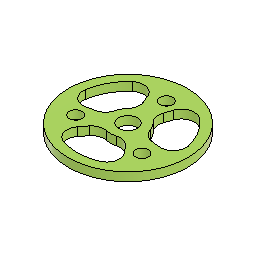
电机2312s磁编码器d4x2定位架 v1 (Autodesk Fusion 360 design; units mm, degrees)
Autodesk Fusion 360 part; units mm, degrees
sketch "草图1" plane through (0, 0, 0) normal (0, 0, 1) x (1, 0, 0)
  circle A0 centre (0, 0) radius 14.1
  line L0 (0, 9.064) -> (-7.85, -4.5326)
  line L1 (-7.85, -4.5326) -> (7.85, -4.5326)
  line L2 (7.85, -4.5326) -> (0, 9.064)
  line L3 (0, 9.064) -> (15.7, 9.064) construction
  circle A1 centre (0, 9.064) radius 1.5
  circle A2 centre (-7.85, -4.5326) radius 1.5
  circle A3 centre (7.85, -4.5326) radius 1.5
  point P0 (0, -0.0004)
  dimension "d1" = 28.2
  dimension "d2" = 15.7
  dimension "d3" = 120
  dimension "d4" = 9.064
  dimension "d5" = 3
  dimension "d6" = 3
  dimension "d7" = 3
  constraint coincident A0.centre origin
  constraint horizontal L3
  constraint coincident L0.start L2.end
  constraint coincident L0.end L1.start
  constraint coincident L1.end L2.start
  measures "d1" diameter of A0
  measures "d2" distance of L0.start L0.end
  measures "d3" angle of L0 L3
  measures "d4" distance of A0.centre L0.start
  measures "d5" diameter of A1
  measures "d6" diameter of A2
  measures "d7" diameter of A3
extrude "拉伸1" add sketch "草图1" along normal blind 2 contours A0 | L0 L1 L2 A1 A2 A3
sketch "草图2" plane through (0, 0, 2) normal (0, 0, 1) x (-1, 0, 0)
  circle A0 centre (7.85, 4.5326) radius 1.5
  circle A1 centre (-7.85, 4.5326) radius 1.5
  circle A2 centre (0, -9.064) radius 1.5
  circle A3 centre (0, 0) radius 14.1
  circle A4 centre (0, 0) radius 2.2
  circle A5 centre (0, 0) radius 12
  circle A6 centre (0, 0) radius 4.2
  line L0 (0, 0) -> (4.5287, -11.1127)
  line L1 (0, 0) -> (11.7731, 2.3225)
  line L2 (0, 0) -> (7.3595, 9.4783)
  line L3 (0, 0) -> (-7.8979, 9.0345)
  line L4 (0, 0) -> (-11.8882, 1.6344)
  line L5 (0, 0) -> (-3.8752, -11.3571)
  dimension "d10" = 4.4
  dimension "d13" = 24
  dimension "d14" = 8.4
  dimension "d16" = 360
  constraint concentric A3 A4
  constraint concentric A4 A5
  constraint concentric A5 A6
  constraint coincident A3.centre A4.centre
  constraint coincident A5 L0.end
  constraint coincident A5 L1.end
  measures "d10" diameter of A4
  measures "d13" diameter of A5
  measures "d14" diameter of A6
extrude "拉伸2" cut sketch "草图2" against normal blind 8 contours A4 L0 L1 | A4 L1 L2 | A4 L0 L5 | A4 L2 L3 | A4 L3 L4 | A4 L4 L5 | A5 A6 L0 L1 | A5 A6 L2 L3 | A5 A6 L4 L5
fillet "圆角1" radius 3 12 edges at (-1.585, 3.8894, 1) (-4.1206, -0.8129, 1) (-2.5758, -3.3174, 1) (2.7643, -3.1621, 1) (4.1609, -0.572, 1) (1.3563, 3.975, 1) (3.8752, 11.3571, 1) (11.8882, -1.6344, 1) (-4.5287, 11.1127, 1) (-11.7731, -2.3225, 1) (-7.3595, -9.4783, 1) (7.8979, -9.0345, 1)
